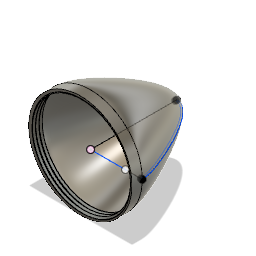
FalconHeavy-PayloadCone (Autodesk Fusion 360 design; units mm, degrees)
Autodesk Fusion 360 part; units mm, degrees
sketch "Sketch1" plane through (0, 0, 0) normal (0, 1, 0) x (1, 0, 0)
  line L0 (0, 0) -> (30, 0)
  line L1 (30, 0) -> (29.2, 0)
  line L2 (0, 0) -> (0, 30)
  line L3 (0, 30) -> (0, 29.2)
  spline S0 degree 5 poles (30, 0) (30, 1.3022) (29.5705, 4.0376) (27.6392, 8.533) (22.9102, 15.0712) (15.0712, 22.9102) (8.533, 27.6392) (4.0376, 29.5705) (1.3022, 30) (0, 30) knots 0 0 0 0 0 0 0.2 0.4 0.6 0.8 1 1 1 1 1 1
  line L4 (2.5, 30) -> (-2.5, 30)
  line L5 (30, -2.5) -> (30, 2.5)
  spline S1 degree 5 poles (29.2, 0) (29.2191, 1.0352) (28.8227, 3.3173) (26.9255, 7.3742) (22.2227, 13.7342) (14.447, 21.7316) (8.051, 26.6713) (3.7541, 28.7153) (1.1996, 29.1871) (0, 29.2) knots 0 0 0 0 0 0 0.2 0.4 0.6 0.8 1 1 1 1 1 1
  line L6 (2.3018, 29.1752) -> (-2.3018, 29.2248)
  line L7 (29.1637, -1.9685) -> (29.2363, 1.9685)
  line L8 (30, 0) -> (30, -6)
  line L9 (29.2, 0) -> (29.2, -6)
  line L10 (30, -6) -> (29.2, -6)
  dimension "d1" = 30
  dimension "d3" = 0.8
  dimension "d4" = 30
  dimension "d5" = 0.8
  dimension "d6" = 6
  dimension "d7" = 6
  dimension "d8" = 0.8
  constraint coincident L0.start L2.start
  constraint horizontal L0
  constraint parallel L0 L1
  constraint vertical L2
  constraint parallel L2 L3
  constraint midpoint L2.end L4
  constraint midpoint L0.end L5
  constraint midpoint L3.end L6
  constraint midpoint L1.end L7
  constraint perpendicular L0 L8
  constraint perpendicular L1 L9
  constraint perpendicular L9 L10
  measures "d1" distance of L0.start L0.end
  measures "d3" distance of L0.end L1.end
  measures "d4" distance of L0.start L2.end
  measures "d5" distance of L2.end L3.end
  measures "d6" distance of L0.end L8.end
  measures "d7" distance of L1.end L9.end
  measures "d8" distance of L8.end L9.end
revolve "Revolve1" add sketch "Sketch1" angle 360 about axis through (0, 0, 0) along (0, 0, -1) contours L0 L1 L5 L8 L9 L10
thread "Thread1" "ISO Metric profile 58.0 M58x2 6H" major diameter 58.2623 minor diameter 56.0224 pitch 2 angle 60 modelled right hand crest width 0.25 on face at (29.1637, 1.4555, 2) crest through (28.0112, 0, -1.125)
sketch "Sketch2" plane through (0, 0, 0) normal (0, 1, 0) x (1, 0, 0)
  line L0 (0, 0) -> (0, 50)
  line L1 (0, 0) -> (30, 0)
  line L2 (30, 0) -> (29.2, 0)
  line L3 (0, 50) -> (0, 49.2)
  spline S0 degree 5 poles (30, 0) (30, 1.2003) (29.593, 4.1779) (27.7628, 10.3737) (23.2662, 21.3333) (15.695, 36.0234) (9.1672, 45.3155) (4.458, 49.1478) (1.4621, 50) (0, 50) knots 0 0 0 0 0 0 0.2 0.4 0.6 0.8 1 1 1 1 1 1
  line L4 (2.1, 50) -> (-2.1, 50)
  line L5 (30, -2) -> (30, 2)
  spline S1 degree 5 poles (29.2, 0) (29.2156, 0.8143) (28.8459, 3.1428) (27.0896, 8.7333) (22.7215, 19.5048) (15.3372, 34.5323) (8.9612, 44.2074) (4.3588, 48.2439) (1.4297, 49.1749) (0, 49.2) knots 0 0 0 0 0 0 0.2 0.4 0.6 0.8 1 1 1 1 1 1
  line L6 (2.0456, 49.1641) -> (-2.0456, 49.2359)
  line L7 (29.1743, -1.341) -> (29.2257, 1.341)
  line L8 (0, 0) -> (21, 0)
  line L9 (21, 0) -> (20.2, 0)
  dimension "d11" = 50
  dimension "d12" = 30
  dimension "d13" = 0.8
  dimension "d14" = 0.8
  dimension "d17" = 21
  dimension "d18" = 0.8
  constraint coincident L0.start L1.start
  constraint vertical L0
  constraint perpendicular L0 L1
  constraint parallel L1 L2
  constraint parallel L0 L3
  constraint midpoint L0.end L4
  constraint midpoint L1.end L5
  constraint midpoint L3.end L6
  constraint midpoint L2.end L7
  constraint parallel L8 L9
  measures "d11" distance of L0.start L0.end
  measures "d12" distance of L0.start L1.end
  measures "d13" distance of L1.end L2.end
  measures "d14" distance of L0.end L3.end
  measures "d17" distance of L8.end L0.start
  measures "d18" distance of L8.end L9.end
revolve "Revolve3" add sketch "Sketch2" angle 360 about axis through (0, 0, 0) along (0, 0, -1) contours L0 L1 L2 L3 S0 S1
revolve "Revolve2" [suppressed]
equation "Wall_Thickness = 0.8 mm"
equation "d3 = Wall_Thickness"
equation "d5 = Wall_Thickness"
equation "d8 = Wall_Thickness"
equation "d13 = Wall_Thickness"
equation "d14 = Wall_Thickness"
equation "d18 = Wall_Thickness"
